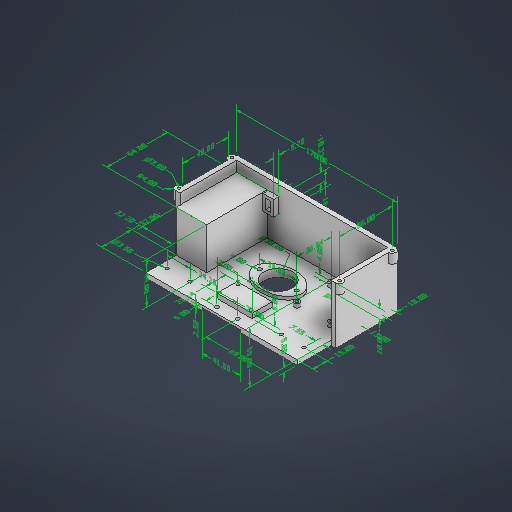
# Autodesk Inventor part: Mitad_2
Saved by Autodesk Inventor 2026.2 (Build 302298000, 298)
## iProperties
Created: 2025-11-05
Part Number: Mitad_2
Material: Genérico
Document SubType Name: Modeling
Designer: 100094631
Density: 1 g/cm^3
Appearance: Valor por defecto
Author: 100094631
Autodesk Inventor part; units mm, degrees
ref_plane "YZ Plane" through (0, 0, 0) normal (1, 0, 0) x (0, 1, 0)
ref_plane "XZ Plane" through (0, 0, 0) normal (0, 1, 0) x (-1, 0, 0)
ref_plane "XY Plane" through (0, 0, 0) normal (0, 0, 1) x (1, 0, 0)
sketch "Boceto1" plane through (0, 0, 0) normal (0, 1, 0) x (-1, 0, 0)
  line L0 (160, -36) -> (165, -36)
  line L1 (165, -36) -> (165, -101)
  line L2 (165, -101) -> (-5, -101)
  line L3 (160, 0) -> (0, 0)
  line L4 (0, 0) -> (0, -36)
  line L5 (0, -36) -> (-5, -36)
  line L6 (-5, -36) -> (-5, -101)
  line L7 (160, 0) -> (160, -36)
  dimension "d250" = 0
  dimension "d4" = 5
  dimension "d5" = 65
  dimension "d87" = 36
  dimension "d88" = 5
  dimension "d89" = 65
  dimension "d132" = 160
  dimension "d301" = 36
  constraints: 16 end point, 4 perpendicular, 2 vertical, 1 horizontal
  measures "d4" distance of L0.start L0.end
  measures "d5" distance of L0.end L1.end
  measures "d87" distance of L3.end L4.end
  measures "d88" distance of L4.end L5.end
  measures "d89" distance of L5.end L2.end
  measures "d132" distance of L3.start L3.end
  measures "d301" distance of L3.start L0.start
extrude "Extrusión1" add sketch "Boceto1" against normal blind 5
sketch "Boceto3" plane through (-160, 0, 0) normal (0, 0, 1) x (1, 0, 0)
  line L0 (0, 0) -> (160, 0) projected
  line L1 (160, -5) -> (0, -5) projected
  line L2 (80, -2.5) -> (80, -5)
  line L3 (160, -5) -> (80, -5)
  line L4 (80, -5) -> (100.5, -5)
  line L5 (100.5, -5) -> (100.5, -2.5)
  line L6 (100.5, -2.5) -> (59.5, -2.5)
  line L7 (59.5, -2.5) -> (59.5, -5)
  line L8 (59.5, -5) -> (80, -5)
  point P0 (100, -5)
  point P1 (60, -5)
  point P2 (165, -5)
  dimension "d140" = 80
  dimension "d410" = 20.5
  dimension "d411" = 2.5
  dimension "d412" = 41
  dimension "d413" = 2.5
  constraints: 14 end point, 2 perpendicular, 2 point on line, 1 collinear, 1 midpoint
  measures "d140" distance of L1.start L3.end
  measures "d410" distance of L3.end L4.end
  measures "d411" distance of L4.end L5.end
  measures "d412" distance of L5.end L6.end
  measures "d413" distance of L6.end L7.end
extrude "Extrusión2" cut sketch "Boceto3" against normal blind 16
sketch "Boceto4" plane through (0, 0, 0) normal (0, 1, 0) x (1, 0, 0)
  circle A0 centre (-7.55, 15) radius 1.75
  circle A1 centre (-31.75, 15) radius 1.75
  circle A2 centre (-152.45, 15) radius 1.75
  circle A3 centre (-128.25, 15) radius 1.75
  line L0 (-140, 0) -> (-140, 36) projected
  line L1 (0, 0) -> (0, 15)
  line L2 (0, 36) -> (0, 0) projected
  line L3 (0, 15) -> (-7.55, 15)
  line L4 (-160, 0) -> (-160, 15)
  line L5 (-160, 0) -> (-160, 36) projected
  line L6 (-160, 15) -> (-152.45, 15)
  line L7 (-152.45, 15) -> (-128.25, 15)
  line L8 (-7.55, 15) -> (-31.75, 15)
  dimension "d16" = 3.5
  dimension "d18" = 3.5
  dimension "d21" = 3.5
  dimension "d23" = 3.5
  dimension "d138" = 15
  dimension "d141" = 7.55
  dimension "d142" = 15
  dimension "d143" = 7.55
  constraints: 4 centre point, 3 horizontal alignment, 3 vertical alignment, 2 end point, 1 horizontal, 14 other
  measures "d16" diameter of A0
  measures "d18" diameter of A1
  measures "d21" diameter of A2
  measures "d23" diameter of A3
  measures "d138" distance of point (0, 0) point (0, 15)
  measures "d141" distance of point (0, 15) L8.start
  measures "d142" distance of point (-160, 0) point (-160, 15)
  measures "d143" distance of point (-160, 15) point (-152.45, 15)
extrude "Extrusión3" cut sketch "Boceto4" against normal blind 5
sketch "Boceto5" plane through (0, 0, 0) normal (0, 1, 0) x (1, 0, 0)
  line L0 (-165, 36) -> (-165, 101)
  line L1 (-165, 101) -> (5, 101)
  line L2 (-165, 36) -> (-160, 36)
  line L3 (-160, 41) -> (-160, 41)
  line L4 (-160, 41) -> (-160, 96)
  line L5 (-160, 96) -> (0.7104, 96)
  line L6 (-160, 41) -> (-160, 36)
  line L7 (-9.2896, 35) -> (-9.2896, 39.9954)
  line L8 (5, 36) -> (5, 101) projected
  line L9 (5, 101) -> (5, 36)
  line L10 (5, 36) -> (0, 36)
  line L11 (0, 36) -> (0, 96)
  point P0 (0, 0)
  point P1 (25, 35)
  dimension "d28" = 5
  constraints: 22 end point, 2 perpendicular, 1 collinear, 1 point on line, 1 vertical, 2 other
  measures "d28" distance between parallel lines of L2 L3
extrude "Extrusión4" add sketch "Boceto5" along normal blind 55
sketch "Boceto10" plane through (0, 0, 0) normal (0, 1, 0) x (1, 0, 0)
  line L0 (0, 0) -> (-80, 0)
  line L1 (0, 0) -> (-160, 0) projected
  line L2 (-80, 0) -> (-80, 60)
  line L3 (-80, 60) -> (-80, 42.5)
  line L4 (-80, 60) -> (-55, 60)
  ellipse E0 centre (-80, 60) end of major axis (-80, 42.5) minor radius 25
  point P0 (-60, 0)
  dimension "d74" = 80
  dimension "d75" = 60
  dimension "d76" = 17.5
  dimension "d77" = 25
  constraints: 8 end point, 1 coincident, 1 collinear, 1 horizontal, 1 perpendicular, 1 point on line, 1 vertical, 4 other
  measures "d74" distance of L0.start L0.end
  measures "d75" distance of L0.end L2.end
  measures "d76" distance of L2.end L3.end
  measures "d77" distance of L2.end L4.end
extrude "Extrusión9" add sketch "Boceto10" along normal blind 3.3
sketch "Boceto11" plane through (0, 3.3, 0) normal (0, 1, 0) x (1, 0, 0)
  ellipse E0 centre (-80, 60) end of major axis (-55, 60) minor radius 17.5 projected
  line L0 (-80, 60) -> (-60.5, 60)
  line L1 (-80, 60) -> (-99.5, 60)
  circle A0 centre (-80, 60) radius 15
  circle A1 centre (-99.5, 60) radius 2
  circle A2 centre (-60.5, 60) radius 2
  line L2 (0, 36) -> (0, 0) projected
  line L3 (-160, 0) -> (0, 0) projected
  dimension "d80" = 19.5
  dimension "d81" = 19.5
  dimension "d82" = 30
  dimension "d83" = 4
  dimension "d84" = 4
  constraints: 4 end point, 3 centre point, 3 coincident, 2 horizontal
  measures "d80" distance of L0.start L0.end
  measures "d81" distance of L0.start L1.end
  measures "d82" diameter of A0
  measures "d83" diameter of A1
  measures "d84" diameter of A2
extrude "Extrusión10" cut sketch "Boceto11" against normal blind 15 contours L1 A0 L0 | L0 A0 L1 | A2 | A1
sketch "Boceto14" plane through (0, 0, 0) normal (0, 1, 0) x (1, 0, 0)
  line L0 (-160, 0) -> (0, 0) projected
  line L1 (-101.57, 13.86) -> (-58.43, 13.86)
  line L2 (-58.43, 35) -> (-101.57, 35)
  line L3 (-101.57, 35) -> (-101.57, 13.86)
  ellipse E0 centre (-80, 60) end of major axis (-55, 60) minor radius 17.5 projected
  line L4 (-58.43, 35) -> (-58.43, 13.86)
  dimension "d328" = 21.14
  dimension "d375" = 43.14
  constraints: 8 end point, 1 horizontal, 1 parallel, 1 vertical
  measures "d328" distance of L2.end L1.start
  measures "d375" distance of L2.start L2.end
extrude "Extrusión13" add sketch "Boceto14" along normal blind 5 contours L3 L2 L4 L1
sketch "Boceto15" plane through (0, 5, 0) normal (0, 1, 0) x (1, 0, 0)
  line L0 (-58.43, 35) -> (-101.57, 35) projected
  line L1 (-101.57, 35) -> (-95.07, 35)
  line L2 (-95.07, 35) -> (-95.07, 32.5)
  line L3 (-58.43, 13.86) -> (-64.93, 13.86)
  line L4 (-64.93, 13.86) -> (-64.93, 16.36)
  circle A0 centre (-95.07, 32.5) radius 1.5
  circle A1 centre (-64.93, 16.36) radius 1.5
  line L5 (-95.07, 32.5) -> (-64.93, 32.5)
  point P0 (0, 0)
  dimension "d158" = 6.5
  dimension "d159" = 2.5
  dimension "d160" = 6.5
  dimension "d161" = 2.5
  dimension "d162" = 3
  dimension "d163" = 3
  constraints: 10 end point, 2 centre point, 2 coincident, 2 perpendicular, 1 horizontal, 1 point on line
  measures "d158" distance of L0.end L1.end
  measures "d159" distance of L1.end L2.end
  measures "d160" distance of L3.start L3.end
  measures "d161" distance of L3.end L4.end
  measures "d162" diameter of A0
  measures "d163" diameter of A1
extrude "Extrusión14" cut sketch "Boceto15" against normal blind 5
sketch "Boceto16" plane through (0, 5, 0) normal (0, 1, 0) x (1, 0, 0)
  line L0 (-58.43, 35) -> (-101.57, 35) projected
  line L1 (-58.43, 35) -> (-61.43, 35)
  line L2 (-61.43, 35) -> (-61.43, 13.86)
  line L3 (-61.43, 13.86) -> (-58.43, 13.86)
  line L4 (-58.43, 13.86) -> (-58.43, 35)
  line L5 (-98.57, 35) -> (-101.57, 35)
  line L6 (-101.57, 35) -> (-101.57, 13.86)
  line L7 (-101.57, 13.86) -> (-98.57, 13.86)
  line L8 (-98.57, 13.86) -> (-98.57, 35)
  point P0 (0, 0)
  dimension "d166" = 3
  dimension "d168" = 21.14
  dimension "d169" = 3
  dimension "d170" = 21.14
  dimension "d374" = 43.14
  constraints: 16 end point, 2 vertical, 1 point on line
  measures "d166" distance of L0.start L1.end
  measures "d168" distance of L1.end L2.end
  measures "d169" distance of L8.end L6.start
  measures "d170" distance of L6.start L6.end
  measures "d374" distance of L0.start L0.end
extrude "Extrusión15" cut sketch "Boceto16" against normal blind 5
sketch "Boceto17" plane through (0, 0, 0) normal (0, 1, 0) x (1, 0, 0)
  line L0 (0, 96) -> (-160, 96) projected
  line L1 (0, 96) -> (0, 86)
  line L2 (0, 36) -> (0, 96) projected
  line L3 (0, 86) -> (-13, 86)
  circle A0 centre (-13, 86) radius 3
  line L4 (-13, 86) -> (-49.54, 86)
  line L5 (-49.54, 86) -> (-49.54, 49.46)
  line L6 (-49.54, 49.46) -> (-13, 49.46)
  line L7 (-13, 49.46) -> (-13, 86)
  circle A1 centre (-49.54, 86) radius 3
  circle A2 centre (-49.54, 49.46) radius 3
  circle A3 centre (-13, 49.46) radius 3
  point P0 (0, 0)
  dimension "d173" = 10
  dimension "d174" = 13
  dimension "d175" = 6
  dimension "d176" = 36.54
  dimension "d177" = 36.54
  dimension "d178" = 36.54
  dimension "d182" = 6
  dimension "d183" = 6
  dimension "d184" = 6
  constraints: 12 end point, 4 centre point, 3 perpendicular, 1 coincident, 1 horizontal, 1 point on line
  measures "d173" distance of L0.start L1.end
  measures "d174" distance of L1.end L3.end
  measures "d175" diameter of A0
  measures "d176" distance of L4.start L4.end
  measures "d177" distance of L4.end L5.end
  measures "d178" distance of L5.end L6.end
  measures "d182" diameter of A1
  measures "d183" diameter of A2
  measures "d184" diameter of A3
extrude "Extrusión16" add sketch "Boceto17" along normal blind 4 contours A0 L7 L3 | L3 L4 A0 | L7 A0 L4 | A1 L5 L4 | L4 L5 A1 | A3 L6 L7 | L7 L6 A3 | A2 L6 L5 | L5 L6 A2
sketch "Boceto18" plane through (-49.54, 4, -86) normal (0, 1, 0) x (1, 0, 0)
  circle A0 centre (0, 0) radius 1.5
  circle A1 centre (36.54, 0) radius 3 projected
  circle A2 centre (36.54, 0) radius 1.5
  circle A3 centre (0, -36.54) radius 3 projected
  circle A4 centre (0, -36.54) radius 1.5
  circle A5 centre (36.54, -36.54) radius 3 projected
  circle A6 centre (36.54, -36.54) radius 1.5
  point P0 (49.54, -86)
  dimension "d187" = 3
  dimension "d188" = 3
  dimension "d189" = 3
  dimension "d190" = 3
  constraints: 4 centre point, 3 coincident
  measures "d187" diameter of A0
  measures "d188" diameter of A2
  measures "d189" diameter of A4
  measures "d190" diameter of A6
extrude "Extrusión17" cut sketch "Boceto18" against normal blind 5 contours A0 | A2 | A4 | A6
sketch "Boceto21" plane through (0, 55, 0) normal (0, 1, 0) x (1, 0, 0)
  circle A0 centre (5, 40) radius 4
  line L0 (-165, 36) -> (-165, 101) projected
  circle A1 centre (-165, 96) radius 4
  circle A2 centre (-165, 40) radius 4
  line L1 (0, 96) -> (-160, 96) projected
  line L2 (0, 96) -> (5, 96)
  circle A3 centre (5, 96) radius 4
  line L3 (-165, 101) -> (-165, 96)
  point P0 (0, 0)
  point P1 (-165, 41.5)
  point P2 (-165, 38.5)
  point P3 (5, 101)
  dimension "d210" = 8
  dimension "d214" = 8
  dimension "d215" = 8
  dimension "d262" = 5
  dimension "d263" = 8
  dimension "d372" = 5
  constraints: 4 centre point, 4 end point, 2 point on line, 1 coincident, 1 horizontal
  measures "d210" diameter of A0
  measures "d214" diameter of A1
  measures "d215" diameter of A2
  measures "d262" distance of L1.start L2.end
  measures "d263" diameter of A3
  measures "d372" distance of L0.end L3.end
extrude "Extrusión18" add sketch "Boceto21" against normal blind 10
sketch "Boceto22" plane through (0, 55, 0) normal (0, 1, 0) x (1, 0, 0)
  arc A0 (5, 36) -> (5, 44) centre (5, 40) ccw projected
  arc A1 (5, 91.0001) -> (5, 98.9999) centre (4.9732, 95) ccw projected
  arc A2 (-165, 100) -> (-165, 92) centre (-165, 96) ccw projected
  circle A3 centre (-165, 96) radius 1.5
  line L0 (-165, 36) -> (-165, 101) projected
  circle A4 centre (-165, 40) radius 1.5
  line L1 (0, 96) -> (0, 36) projected
  circle A5 centre (5, 96) radius 1.5
  line L2 (5, 40) -> (0, 40)
  line L3 (0, 36) -> (0, 40)
  circle A6 centre (5, 40) radius 1.5
  line L4 (0, 96) -> (5, 96)
  line L5 (-160, 96) -> (-160, 36) projected
  point P0 (0, 0)
  dimension "d218" = 3
  dimension "d219" = 3
  dimension "d259" = 3
  dimension "d260" = 5
  dimension "d261" = 3
  constraints: 6 end point, 4 centre point, 2 coincident, 2 horizontal, 2 point on line, 1 vertical
  measures "d218" diameter of A3
  measures "d219" diameter of A4
  measures "d259" diameter of A5
  measures "d260" distance of L2.start L2.end
  measures "d261" diameter of A6
extrude "Extrusión19" cut sketch "Boceto22" against normal blind 5 contours A4 L0 | L0 A4 | L0 A3 | A3 L0 | A6 | A5
sketch "Boceto24" plane through (-160, 0, -96) normal (0, 0, 1) x (1, 0, 0)
  line L0 (0, 55) -> (160, 55) projected
  line L1 (29.2, 0) -> (0, 0)
  line L2 (0, 0) -> (29.2, 0)
  line L3 (0, 0) -> (0, -5) projected
  line L4 (0, 0) -> (0, 41)
  line L5 (0, 0) -> (0, 55) projected
  line L6 (0, 41) -> (29.2, 41)
  line L7 (29.2, 41) -> (29.2, 0)
  line L8 (29.2, 0) -> (0, 0)
  line L9 (32.2, 44) -> (-3, 44)
  line L10 (-3, 44) -> (-3, -3)
  line L11 (-3, -3) -> (32.2, -3)
  line L12 (32.2, -3) -> (32.2, 44)
  line L13 (29.2, 0) -> (29.2, 10)
  line L14 (29.2, 10) -> (0, 10)
  point P0 (160, 0)
  point P1 (0, 10)
  point P2 (0, 44)
  point P3 (0, -3)
  dimension "d243" = 41
  dimension "d244" = 29.2
  dimension "d246" = 3
  dimension "d247" = 10
  dimension "d248" = 29.2
  constraints: 24 end point, 3 point on line, 2 collinear, 2 perpendicular, 1 vertical, 3 other
  measures "d243" distance of L1.end L4.end
  measures "d244" distance of L4.end L6.end
  measures "d246" distance between parallel lines of L6 L9
  measures "d247" distance of L1.start L13.end
  measures "d248" distance of L13.end L14.end
extrude "Extrusión21" cut sketch "Boceto24" against normal blind 10 contours L14 L4 L6 L7
extrude "Extrusión22" add sketch "Boceto24" along normal blind 61 contours L7 L6 L5 L9 L12 L11 L3 L1
sketch "Boceto25" plane through (-160, 44, -96) normal (0, 1, 0) x (1, 0, 0)
  line L0 (0, -96) -> (0, -60) projected
  line L1 (0, -61) -> (0, -64)
  line L2 (0, -64) -> (32.2, -64)
  line L3 (32.2, -64) -> (32.2, -61)
  line L4 (32.2, -61) -> (0, -61)
  point P0 (160, -96)
  point P1 (0, -61)
  constraints: 8 end point, 2 perpendicular, 1 horizontal, 1 point on line
extrude "Extrusión23" add sketch "Boceto25" against normal blind 44
sketch "Boceto26" plane through (5, -5, -101) normal (0, 0, -1) x (-1, 0, 0)
  line L0 (125.8, 46) -> (125.8, 31)
  line L1 (125.8, 31) -> (120.8, 31)
  line L2 (132.8, 49) -> (132.8, 5) projected
  line L3 (120.8, 31) -> (130.8, 31)
  line L4 (130.8, 31) -> (130.8, 13)
  line L5 (130.8, 13) -> (120.8, 13)
  line L6 (120.8, 13) -> (120.8, 31)
  line L7 (135.8, 46) -> (135.8, 5) projected
  line L8 (125.8, 46) -> (135.8, 46)
  point P0 (5, 5)
  dimension "d277" = 15
  dimension "d278" = 5
  dimension "d280" = 18
  dimension "d281" = 10
  constraints: 14 end point, 4 perpendicular, 1 horizontal, 1 vertical
  measures "d277" distance of L0.start L0.end
  measures "d278" distance of L0.end L1.end
  measures "d280" distance of L3.end L4.end
  measures "d281" distance of L4.end L5.end
extrude "Extrusión24" add sketch "Boceto26" along normal blind 12
sketch "Boceto28" plane through (-125.8, 8, -101) normal (-1, 0, 0) x (0, 0, 1)
  line L0 (-12, 0) -> (-12, 9)
  line L1 (-12, 0) -> (-12, 18) projected
  line L2 (-12, 9) -> (-6, 9)
  line L3 (-9.5, 1.5) -> (-2.5, 1.5)
  line L4 (-2.5, 1.5) -> (-2.5, 16.5)
  line L5 (-2.5, 16.5) -> (-9.5, 16.5)
  line L6 (-9.5, 16.5) -> (-9.5, 1.5)
  point P0 (101, -8)
  dimension "d293" = 9
  dimension "d294" = 6
  dimension "d297" = 7
  dimension "d298" = 15
  constraints: 12 end point, 2 parallel, 2 perpendicular, 1 horizontal, 1 midpoint
  measures "d293" distance of L0.start L0.end
  measures "d294" distance of L0.end L2.end
  measures "d297" distance of L5.end L4.end
  measures "d298" distance of L4.end L3.end
extrude "Extrusión25" cut sketch "Boceto28" against normal blind 10
sketch "Boceto31" plane through (0, 0, 0) normal (0, 1, 0) x (1, 0, 0)
  circle A0 centre (-69, 6) radius 2
  circle A1 centre (-91, 6) radius 2
  line L0 (-91, 6) -> (-69, 6)
  line L1 (-80, 0) -> (-80, 6)
  point P0 (0, 0)
  dimension "d368" = 4
  dimension "d369" = 4
  dimension "d376" = 6
  constraints: 4 end point, 2 centre point, 1 horizontal, 1 midpoint, 1 vertical
  measures "d368" diameter of A0
  measures "d369" diameter of A1
  measures "d376" distance of L1.start L1.end
extrude "Extrusión30" cut sketch "Boceto31" against normal blind 5
sketch "Boceto33" plane through (5, -5, -101) normal (0, 0, -1) x (-1, 0, 0)
  line L0 (120.8, 31) -> (130.8, 31) projected
  line L1 (125.8, 31) -> (125.8, 36)
  line L2 (125.8, 36) -> (123.19, 36)
  line L3 (125.8, 36) -> (128.41, 36)
  line L4 (128.41, 36) -> (128.41, 46.22)
  line L5 (128.41, 46.22) -> (123.19, 46.22)
  line L6 (123.19, 46.22) -> (123.19, 36)
  line L7 (120.19, 49.22) -> (131.41, 49.22)
  line L8 (131.41, 49.22) -> (131.41, 33)
  line L9 (131.41, 33) -> (125.8, 33)
  line L10 (125.8, 33) -> (120.19, 33)
  line L11 (120.19, 33) -> (120.19, 49.22)
  point P0 (5, 5)
  dimension "d387" = 5
  dimension "d388" = 2.61
  dimension "d389" = 2.61
  dimension "d390" = 10.22
  dimension "d391" = 5.22
  dimension "d394" = 3
  constraints: 22 end point, 2 horizontal, 2 perpendicular, 2 vertical, 1 midpoint, 4 other
  measures "d387" distance of L1.start L1.end
  measures "d388" distance of L1.end L2.end
  measures "d389" distance of L1.end L3.end
  measures "d390" distance of L3.end L4.end
  measures "d391" distance of L4.end L5.end
  measures "d394" distance between parallel lines of L5 L7
extrude "Extrusión34" add sketch "Boceto33" against normal blind 10.7
extrude "Extrusión35" cut sketch "Boceto33" against normal blind 8.7 contours L2 L6 L5 L4 L3
